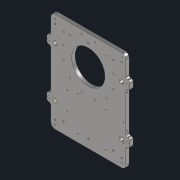
# Autodesk Inventor part: base5
Saved by Autodesk Inventor 2021 (Build 250183000, 183)
## iProperties
Created: 2021-07-20
Part Number: base5
Material: 鋼、炭素鋼
Document SubType Name: モデリング
Designer: yuta0
Density: 7.85 g/cm^3
Appearance: 半つや出し
Sheet Metal Rule: Default_mm
Mass: 2468.64 g
Surface Area: 925.307 cm^2
Volume: 314.476 cm^3
購入先: Meviy
在庫数: 0.0
Author: yuta0
Autodesk Inventor part; units mm, degrees
ref_plane "YZ Plane" through (0, 0, 0) normal (1, 0, 0) x (0, 1, 0)
ref_plane "XZ Plane" through (0, 0, 0) normal (0, 1, 0) x (-1, 0, 0)
ref_plane "XY Plane" through (0, 0, 0) normal (0, 0, 1) x (1, 0, 0)
sketch "スケッチ1" plane through (0, 0, 0) normal (0, 0, 1) x (1, 0, 0)
  circle A0 centre (0, 0) radius 73.5 construction
  line L0 (-90, -170) -> (90, -170)
  line L1 (90, -170) -> (90, 70)
  line L2 (90, 70) -> (-90, 70)
  line L3 (-90, 70) -> (-90, -170)
  line L4 (-90, -170) -> (90, 70) construction
  line L5 (90, -170) -> (-90, 70) construction
  point P0 (0, -50)
  point P1 (0, -50)
  dimension "d25" = 147
  dimension "d26" = 240
  dimension "d71" = 180
  dimension "d76" = 70
  constraints: 12 end point, 3 midpoint, 2 parallel, 1 centre point, 1 coincident, 1 horizontal, 1 perpendicular, 1 vertical alignment
  measures "d25" diameter of A0
  measures "d26" distance of L0.end L1.end
  measures "d71" distance of L1.end L2.end
  measures "d76" distance from line of point (0, 0) L2
extrude "押し出し2" add sketch "スケッチ1" along normal mid plane 8
sketch "スケッチ5" plane through (0, 0, 4) normal (0, 0, 1) x (1, 0, 0)
  line L0 (-50.5, -116.75) -> (85, -116.75)
  line L1 (85, -116.75) -> (85, -73.25)
  line L2 (85, -73.25) -> (-50.5, -73.25)
  line L3 (-50.5, -73.25) -> (-50.5, -116.75)
  line L4 (-50.5, -116.75) -> (85, -73.25) construction
  line L5 (85, -116.75) -> (-50.5, -73.25) construction
  line L6 (90, -170) -> (90, 70) projected
  point P0 (0, 0)
  point P1 (17.25, -95)
  point P2 (17.25, -95)
  dimension "d40" = 135.5
  dimension "d41" = 43.5
  dimension "d73" = 95
  dimension "d74" = 5
  constraints: 12 end point, 3 midpoint, 2 parallel, 1 horizontal, 1 perpendicular
  measures "d40" distance of L1.end L2.end
  measures "d41" distance of L2.end L0.start
  measures "d73" vertical distance of point (0, 0) point (17.25, -95)
  measures "d74" distance between parallel lines of L6 L1
hole "穴3" at (-50.5, -73.25, 4) at (-50.5, -116.75, 4) at (85, -116.75, 4) at (85, -73.25, 4) direction (0, 0, -1) diameter 2.459 depth 8.8 tip angle 118 thread size "M3x0.5" class "6H" standard "ANSI Metric M Profile"
sketch "スケッチ6" plane through (0, 0, -4) normal (0, 0, -1) x (-1, 0, 0)
  circle A0 centre (0, 0) radius 40
  dimension "d54" = 80
  constraints: 1 centre point, 1 coincident
  measures "d54" diameter of A0
extrude "押し出し3" cut sketch "スケッチ6" against normal through all
sketch "スケッチ7" plane through (0, 0, 4) normal (0, 0, 1) x (1, 0, 0)
  line L0 (-25, -68) -> (42, -68)
  line L1 (42, -68) -> (42, -152)
  line L2 (42, -152) -> (-25, -152)
  line L3 (-25, -152) -> (-25, -68)
  line L4 (-25, -68) -> (42, -152) construction
  line L5 (42, -68) -> (-25, -152) construction
  line L6 (-90, -170) -> (90, -170) projected
  line L7 (-90, 70) -> (-90, -170) projected
  line L8 (90, -170) -> (90, 70) projected
  point P0 (0, 0)
  point P1 (8.5, -110)
  point P2 (-80, -170)
  point P3 (80, -170)
  point P4 (-90, 60)
  point P5 (-90, -160)
  point P6 (90, -160)
  point P7 (90, 60)
  dimension "d59" = 67
  dimension "d60" = 84
  dimension "d70" = 110
  dimension "d75" = 48
  constraints: 12 end point, 2 midpoint, 2 parallel, 1 horizontal, 1 perpendicular
  measures "d59" distance of L1.end L2.end
  measures "d60" distance of L0.end L1.end
  measures "d70" vertical distance of point (0, 0) point (8.5, -110)
  measures "d75" distance between parallel lines of L8 L1
hole "穴4" at (-25, -152, 4) at (-25, -68, 4) at (42, -68, 4) at (42, -152, 4) direction (0, 0, -1) diameter 2.459 depth 8.8 tip angle 118 thread size "M3x0.5" class "6H" standard "ANSI Metric M Profile"
sketch "スケッチ8" plane through (0, 0, -4) normal (0, 0, -1) x (-1, 0, 0)
  point P0 (0, 0)
  point P1 (-80, 60)
  point P2 (80, 60)
  point P3 (80, -160)
  point P4 (-80, -160)
  dimension "d148" = 60
  dimension "d149" = 160
  dimension "d150" = 80
  dimension "d151" = 80
  constraints: 2 horizontal alignment, 2 vertical alignment
  measures "d148" vertical distance of point (0, 0) point (-80, 60)
  measures "d149" vertical distance of point (-80, -160) point (0, 0)
  measures "d150" horizontal distance of point (-80, 60) point (0, 0)
  measures "d151" horizontal distance of point (80, 60) point (0, 0)
hole "穴5" at (80, -160, -4) at (-80, -160, -4) at (-80, 60, -4) at (80, 60, -4) direction (0, 0, 1) diameter 3.2 end through all counterbore diameter 6.5 counterbore depth 3 clearance for "Socket Head Cap Screw" size "M3" standard "Ansi Metric M Profile"
sketch "スケッチ9" plane through (0, 0, 4) normal (0, 0, 1) x (1, 0, 0)
  line L0 (-90, -170) -> (90, -170) projected
  line L1 (90, 70) -> (-90, 70) projected
  point P0 (0, 0)
  point P1 (-60, -144)
  point P2 (60, -144)
  point P3 (-80, -170)
  point P4 (80, -170)
  point P5 (-60, 44)
  point P6 (60, 44)
  point P7 (80, 70)
  point P8 (-80, 70)
  dimension "d84" = 60
  dimension "d85" = 60
  dimension "d86" = 26
  dimension "d94" = 26
  constraints: 2 horizontal alignment, 2 vertical alignment
  measures "d84" horizontal distance of point (0, 0) point (-60, -144)
  measures "d85" horizontal distance of point (60, -144) point (0, 0)
  measures "d86" distance from line of L0 point (-60, -144)
  measures "d94" distance from line of L1 point (-60, 44)
hole "穴6" at (-60, -144, 4) at (60, -144, 4) at (-60, 44, 4) at (60, 44, 4) direction (0, 0, -1) diameter 4.134 end through all thread size "M5x0.8" class "6H" standard "ANSI Metric M Profile"
sketch "スケッチ3" plane through (0, 0, -4) normal (0, 0, 1) x (1, 0, 0)
  circle A0 centre (0, 0) radius 62.5
  point P0 (-16.1762, 60.3704)
  point P1 (-44.1942, 44.1942)
  point P2 (-60.3704, 16.1762)
  point P3 (-60.3704, -16.1762)
  point P4 (-44.1942, -44.1942)
  point P5 (-16.1762, -60.3704)
  point P6 (16.1762, -60.3704)
  point P7 (44.1942, -44.1942)
  point P8 (60.3704, -16.1762)
  point P9 (60.3704, 16.1762)
  point P10 (44.1942, 44.1942)
  point P11 (16.1762, 60.3704)
  dimension "d8" = 125
  dimension "d11" = 360
  dimension "d20" = 0
  constraints: 1 coincident, 16 other
  measures "d20" vertical distance of point (16.176, 60.37) point (-16.176, 60.37)
hole "穴1" at (-16.1762, 60.3704, -4) at (-44.1942, 44.1942, -4) at (-60.3704, 16.1762, -4) at (-60.3704, -16.1762, -4) at (-44.1942, -44.1942, -4) at (-16.1762, -60.3704, -4) at (16.1762, -60.3704, -4) at (44.1942, -44.1942, -4) at (60.3704, -16.1762, -4) at (60.3704, 16.1762, -4) at (44.1942, 44.1942, -4) at (16.1762, 60.3704, -4) direction (0, 0, 1) diameter 4.3 end through all counterbore diameter 8 counterbore depth 4.5 clearance for "Socket Head Cap Screw" size "M4" standard "Ansi Metric M Profile"
sketch "スケッチ4" plane through (0, 0, 4) normal (0, 0, 1) x (1, 0, 0)
  line L0 (-80, -150) -> (80, -150)
  line L1 (80, -150) -> (80, 50)
  line L2 (80, 50) -> (-80, 50)
  line L3 (-80, 50) -> (-80, -150)
  line L4 (-80, -150) -> (80, 50) construction
  line L5 (80, -150) -> (-80, 50) construction
  line L6 (90, 70) -> (-90, 70) projected
  line L7 (-90, -170) -> (90, -170) projected
  line L8 (79.8007, -110) -> (-79.8007, -110)
  line L9 (-79.8007, -110) -> (-79.8007, 10)
  line L10 (-79.8007, 10) -> (79.8007, 10)
  line L11 (79.8007, 10) -> (79.8007, -110)
  line L12 (79.8007, -110) -> (-79.8007, 10) construction
  line L13 (-79.8007, -110) -> (79.8007, 10) construction
  line L14 (40, -150) -> (-40, -150)
  line L15 (-40, -150) -> (-40, 50)
  line L16 (-40, 50) -> (40, 50)
  line L17 (40, 50) -> (40, -150)
  line L18 (40, -150) -> (-40, 50) construction
  line L19 (-40, -150) -> (40, 50) construction
  line L20 (79.6443, -70) -> (-79.6443, -70)
  line L21 (-79.6443, -70) -> (-79.6443, -30)
  line L22 (-79.6443, -30) -> (79.6443, -30)
  line L23 (79.6443, -30) -> (79.6443, -70)
  line L24 (79.6443, -70) -> (-79.6443, -30) construction
  line L25 (-79.6443, -70) -> (79.6443, -30) construction
  line L26 (0, 50) -> (0, -150)
  point P0 (0, 0)
  point P1 (0, -50)
  point P2 (0, -50)
  point P3 (60, 72.5)
  point P4 (-60, 72.5)
  point P5 (-90, 70)
  dimension "d30" = 160
  dimension "d31" = 200
  dimension "d72" = 20
  dimension "d96" = 40
  dimension "d97" = 40
  dimension "d98" = 40
  constraints: 50 end point, 11 midpoint, 8 parallel, 4 horizontal, 4 perpendicular, 1 point on line, 1 vertical alignment, 1 other
  measures "d30" distance of L2.end L1.end
  measures "d31" distance of L1.end L0.end
  measures "d72" distance between parallel lines of L7 L0
  measures "d96" distance between parallel lines of L2 L10
  measures "d97" distance between parallel lines of L10 L22
  measures "d98" distance between parallel lines of L3 L15
hole "穴2" at (80, 50, 4) at (-80, 50, 4) at (-80, -150, 4) at (80, -150, 4) at (0, 50, 4) at (0, -150, 4) direction (0, 0, -1) diameter 4.134 end through all thread size "M5x0.8" class "6H" standard "ANSI Metric M Profile"
sketch "スケッチ10" plane through (-90, -160, 4) normal (-1, 0, 0) x (0, 0, 1)
  line L0 (-8, -10) -> (-8, 230)
  line L1 (-8, -10) -> (-8, 230) projected
  line L2 (-8, 230) -> (0, 230) projected
  line L3 (0, 230) -> (0, -10) projected
  point P0 (-4, 150)
  point P1 (-4, 70)
  dimension "d102" = 80
  dimension "d152" = 80
  constraints: 2 end point, 1 vertical, 1 other
  measures "d102" distance of point (-4, 150) point (-4, 70)
  measures "d152" distance from line of L2 point (-4, 150)
hole "穴7" at (-90, -10, 0) at (-90, -90, 0) direction (1, 0, 0) diameter 2.459 depth 8.8 tip angle 118 thread size "M3x0.5" class "6H" standard "ANSI Metric M Profile"
sketch "スケッチ12" plane through (0, 0, -4) normal (0, 0, -1) x (-1, 0, 0)
  circle A0 centre (80, 50) radius 2.067 projected
  line L0 (90, -170) -> (90, 70) projected
  line L1 (90, 70) -> (-90, 70) projected
  point P0 (0, 0)
  point P1 (90, -160)
  point P2 (90, 60)
  point P3 (80, 70)
  point P4 (-80, 70)
  point P5 (80, 10)
  point P6 (80, -30)
  point P7 (80, -70)
  point P8 (80, -110)
  point P9 (80, -150)
  point P10 (40, 50)
  point P11 (40, 10)
  point P12 (40, -30)
  point P13 (40, -70)
  point P14 (40, -110)
  point P15 (40, -150)
  point P16 (0, 50)
  point P17 (0, 10)
  point P18 (0, -30)
  point P19 (0, -70)
  point P20 (0, -110)
  point P21 (0, -150)
  point P22 (-40, 50)
  point P23 (-40, 10)
  point P24 (-40, -30)
  point P25 (-40, -70)
  point P26 (-40, -110)
  point P27 (-40, -150)
  point P28 (-80, 50)
  point P29 (-80, 10)
  point P30 (-80, -30)
  point P31 (-80, -70)
  point P32 (-80, -110)
  point P33 (-80, -150)
  dimension "d131" = 40
  dimension "d134" = 40
  constraints: 1 horizontal, 1 vertical, 29 other
  measures "d131" distance of A0.centre point (80, 10)
  measures "d134" distance of A0.centre point (40, 50)
hole "穴9" at (-80, 10, -4) at (80, 10, -4) at (-80, -110, -4) at (80, -110, -4) direction (0, 0, 1) diameter 6.4 end through all counterbore diameter 11 counterbore depth 12 clearance for "Socket Head Cap Screw" size "M6" standard "Ansi Metric M Profile"
mirror "ミラー2" about plane through (0, 0, 0) normal (1, 0, 0) of "穴7"
sketch "スケッチ15" plane through (0, 0, 4) normal (0, 0, 1) x (1, 0, 0)
  line L0 (90, 70) -> (-90, 70) projected
  line L1 (90, -170) -> (90, 70) projected
  line L2 (90, 20) -> (100, 20)
  line L3 (100, 20) -> (100, 0)
  line L4 (100, 0) -> (90, 0)
  line L5 (90, 0) -> (90, 20)
  circle A0 centre (80, 10) radius 5.5 projected
  point P0 (0, 0)
  dimension "d173" = 10
  dimension "d174" = 10
  dimension "d175" = 10
  constraints: 8 end point, 2 parallel, 1 horizontal, 1 perpendicular, 1 point on line
  measures "d173" distance between parallel lines of L1 L3
  measures "d174" distance from line of L2 A0.centre
  measures "d175" distance from line of L4 A0.centre
extrude "押し出し4" add sketch "スケッチ15" against normal up to surface (8 mm away) contours L1 L2 L3 L4
sketch "スケッチ16" plane through (0, 0, 4) normal (0, 0, 1) x (1, 0, 0)
  line L0 (90, -170) -> (90, 70) projected
  line L1 (100, 0) -> (100, 20) projected
  line L2 (100, 20) -> (90, 20) projected
  point P0 (0, 0)
  point P1 (95, 10)
  dimension "d176" = 5
  dimension "d177" = 10
  measures "d176" distance from line of L1 point (95, 10)
  measures "d177" distance from line of L2 point (95, 10)
hole "穴10" at (95, 10, 4) direction (0, 0, -1) diameter 5.3 end through all clearance for "Socket Head Cap Screw" size "M5" standard "Ansi Metric M Profile"
mirror "ミラー3" about plane through (0, 0, 0) normal (1, 0, 0) of "押し出し4", "穴10"
fillet "フィレット6" radius 10 4 edges at (90, 70, 0) (-90, 70, 0) (-90, -170, 0) (90, -170, 0)
ref_plane "作業平面4" through (-80, -50, 4) normal (0, 1, 0) x (1, 0, 0)
mirror "ミラー4" about plane through (-80, -50, 4) normal (0, 1, 0) of "押し出し4", "穴10", "ミラー3"
fillet "フィレット7" radius 5 16 edges at (90, 20, 0) (100, 20, 0) (100, 0, 0) (90, 0, 0) (90, -100, 0) (100, -100, 0) (100, -120, 0) (90, -120, 0) (-90, -120, 0) (-100, -120, 0) (-100, -100, 0) (-90, -100, 0) (-90, 0, 0) (-100, 0, 0) (-100, 20, 0) (-90, 20, 0)
equation "\"d82\" = Thickness"
equation "\"d18\" = Thickness"
equation "\"BendRadius\" = Thickness"
equation "\"BendReliefWidth\" = Thickness"
equation "\"BendReliefDepth\" = 0.5 * Thickness"
equation "\"CornerReliefSize\" = 4 * Thickness"
equation "\"MinimumRemnant\" = 2 * Thickness"
equation "\"TransitionRadius\" = BendRadius"
equation "\"JacobiRadiusSize\" = BendRadius"
equation "\"GapSize\" = Thickness"
equation "\"d2\" = Thickness"
equation "\"Thickness\" = 3.2"
